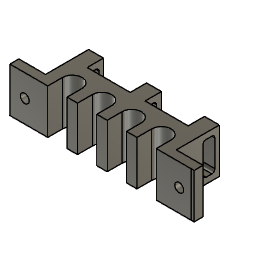
WireClip (Autodesk Fusion 360 design; units mm, degrees)
Autodesk Fusion 360 part; units mm, degrees
sketch "Sketch1" plane through (0, 0, 0) normal (0, 0, 1) x (1, 0, 0)
  line L0 (0, 0) -> (-8, 0)
  line L1 (0, 0) -> (52, 0)
  line L2 (0, 10) -> (44, 10)
  line L3 (44, 10) -> (44, 2)
  line L4 (44, 2) -> (52.000001, 2)
  line L5 (52.000001, 2) -> (52, 0)
  line L6 (-8, 0) -> (-8, 2)
  line L7 (-8, 2) -> (0, 2)
  line L8 (0, 2) -> (0, 10)
  circle A0 centre (7, 5) radius 3.25
  circle A1 centre (17, 5) radius 3.25
  circle A2 centre (37.000001, 5) radius 3.25
  circle A3 centre (27, 5) radius 3.25
  line L9 (7, 5) -> (10.25, 5)
  line L10 (10.25, 5) -> (10.25, -1.628817)
  line L11 (10.25, -1.628817) -> (7, -1.628817)
  line L12 (7, -1.628817) -> (7, 5)
  line L13 (7, 5) -> (3.75, 5)
  line L14 (3.75, 5) -> (3.75, -1.5)
  line L15 (3.75, -1.5) -> (7, -1.5)
  line L16 (7, -1.5) -> (7, 5)
  line L17 (17, 5) -> (20.25, 5)
  line L18 (20.25, 5) -> (20.25, -2)
  line L19 (20.25, -2) -> (17, -2)
  line L20 (17, -2) -> (17, 5)
  line L21 (17, 5) -> (13.75, 5)
  line L22 (13.75, 5) -> (13.75, -3.5)
  line L23 (13.75, -3.5) -> (17, -3.5)
  line L24 (17, -3.5) -> (17, 5)
  line L25 (27, 5) -> (23.75, 5)
  line L26 (23.75, 5) -> (23.75, -2.5)
  line L27 (23.75, -2.5) -> (27, -2.5)
  line L28 (27, -2.5) -> (27, 5)
  line L29 (27, 5) -> (30.25, 5)
  line L30 (30.25, 5) -> (30.25, -3.5)
  line L31 (30.25, -3.5) -> (27, -3.5)
  line L32 (27, -3.5) -> (27, 5)
  line L33 (37.000001, 5) -> (33.750001, 5)
  line L34 (33.750001, 5) -> (33.750001, -1.5)
  line L35 (33.750001, -1.5) -> (37.000001, -1.5)
  line L36 (37.000001, -1.5) -> (37.000001, 5)
  line L37 (37.000001, 5) -> (40.250001, 5)
  line L38 (40.250001, 5) -> (40.250001, -2.5)
  line L39 (40.250001, -2.5) -> (37.000001, -2.5)
  line L40 (37.000001, -2.5) -> (37.000001, 5)
  dimension "d2" = 44
  dimension "d3" = 6.5
  dimension "d4" = 6.5
  dimension "d5" = 6.5
  dimension "d6" = 6.5
  dimension "d9" = 3.25
  dimension "d10" = 3.25
  dimension "d11" = 3.25
  dimension "d12" = 3.25
  constraint coincident L0.start L1.start
  constraint perpendicular L2 L3
  constraint perpendicular L3 L4
  constraint perpendicular L0 L6
  constraint perpendicular L2 L8
  constraint horizontal L9
  constraint vertical L10
  constraint horizontal L11
  constraint vertical L12
  constraint coincident A0.centre L9.start
  constraint horizontal L13
  constraint vertical L14
  constraint horizontal L15
  constraint vertical L16
  constraint horizontal L17
  constraint vertical L18
  constraint horizontal L19
  constraint vertical L20
  constraint coincident A1.centre L17.start
  constraint horizontal L21
  constraint vertical L22
  constraint horizontal L23
  constraint vertical L24
  constraint horizontal L25
  constraint vertical L26
  constraint horizontal L27
  constraint vertical L28
  constraint coincident A3.centre L25.start
  constraint horizontal L29
  constraint vertical L30
  constraint horizontal L31
  constraint vertical L32
  constraint horizontal L33
  constraint vertical L34
  constraint horizontal L35
  constraint vertical L36
  constraint horizontal L37
  constraint vertical L38
  constraint horizontal L39
  constraint vertical L40
  measures "d2" distance of L2.start L2.end
  measures "d3" diameter of A0
  measures "d4" diameter of A1
  measures "d5" diameter of A2
  measures "d6" diameter of A3
  measures "d9" distance of A0.centre L9.end
  measures "d10" distance of A1.centre L17.end
  measures "d11" distance of A3.centre L25.end
sketch "Sketch2" plane through (0, 0, 0) normal (0, 0, 1) x (1, 0, 0)
extrude "Extrude1" add sketch "Sketch1" along normal blind 15 contours L0 L1 L2 L3 L4 L5 L6 L7 L8 A0 A1 A2 A3 L10 L14 L18 L22 L26 L30 L34 L38 picked at (1.2621, 5.828129)
sketch "Sketch3" plane through (0, 2, 0) normal (0, 1, 0) x (-1, 0, 0)
  line L0 (0, 0) -> (8, 0)
  line L1 (8, 0) -> (8, 15)
  line L2 (8, 15) -> (0, 15)
  line L3 (0, 15) -> (0, 0)
  circle A0 centre (4, 7.5) radius 1.5
  circle A1 centre (-48.000001, 7.5) radius 1.5
  dimension "d15" = 3
  dimension "d16" = 3
  measures "d15" diameter of A0
  measures "d16" diameter of A1
extrude "Extrude2" cut sketch "Sketch3" against normal blind 4 contours A0 | A1 picked at (4.091709, 7.857751) picked at (-48.372111, 7.765565)
sketch "Sketch4" plane through (0, 10, 0) normal (0, 1, 0) x (-1, 0, 0)
  line L0 (-44, 0) -> (0, 0)
  line L1 (0, 0) -> (0, 15)
  line L2 (0, 15) -> (-44, 15)
  line L3 (-44, 15) -> (-44, 0)
  line L4 (-5, 0) -> (-5, 15)
  line L5 (-39.000001, 0) -> (-39.000001, 15)
  line L6 (-22, 0) -> (-22, 15)
  line L7 (-22, 12.987575) -> (-19.5, 12.987575)
  line L8 (-19.5, 12.987575) -> (-24.5, 12.987575)
  line L9 (-19.5, 12.987575) -> (-19.5, 15)
  line L10 (-24.5, 12.987575) -> (-24.5, 15)
  line L11 (-19.5, 0) -> (-19.5, 2)
  line L12 (-19.5, 2) -> (-24.5, 2)
  line L13 (-24.5, 2) -> (-24.5, 0)
  line L14 (-5, 12.987575) -> (0, 12.987575)
  line L15 (-5, 2) -> (0, 2)
  line L16 (-39.000001, 13) -> (-44, 13)
  line L17 (-39.000001, 2) -> (-44, 2)
  dimension "d19" = 2.5
  dimension "d20" = 5
  constraint coincident L0 L4.start
  constraint coincident L2 L4.end
  constraint perpendicular L2 L4
  constraint perpendicular L2 L5
  constraint midpoint L0 L6.start
  constraint midpoint L2 L6.end
  constraint perpendicular L6 L7
  constraint perpendicular L6 L8
  constraint coincident L2 L9.end
  constraint perpendicular L2 L9
  constraint coincident L2 L10.end
  constraint perpendicular L2 L10
  constraint coincident L0 L11.start
  constraint perpendicular L0 L11
  constraint perpendicular L6 L12
  constraint coincident L0 L13.end
  constraint perpendicular L12 L13
  constraint perpendicular L1 L14
  constraint coincident L4 L15.start
  constraint coincident L1 L15.end
  constraint perpendicular L1 L15
  constraint coincident L3 L16.end
  constraint perpendicular L3 L16
  constraint coincident L3 L17.end
  constraint perpendicular L3 L17
extrude "Extrude3" add sketch "Sketch4" along normal blind 5 contours L0 L3 L5 L17 | L0 L6 L12 L13 | L2 L3 L5 L16 | L0 L6 L11 L12 | L0 L1 L4 L15 | L2 L6 L8 L10 | L2 L6 L7 L8 L9 | L1 L2 L4 L14 picked at (-42.333334, 1.333333) picked at (-23.666667, 1.333333) picked at (-42.333334, 14.333333) picked at (-21.166667, 1.333333) picked at (-3.333333, 1.333333) picked at (-22.833333, 13.658384) picked at (-21.166667, 14.329192) picked at (-3.333333, 14.329192)
sketch "Sketch5" plane through (0, 0, 12.987575) normal (0, 0, -1) x (1, 0, 0)
  line L0 (24.5, -10) -> (19.5, -10)
  line L1 (19.5, -10) -> (19.5, -15)
  line L2 (19.5, -15) -> (24.5, -15)
  line L3 (24.5, -15) -> (24.5, -10)
  line L4 (24.5, -12.931425) -> (19.5, -12.931425)
  line L5 (5, -10) -> (5, -15)
  line L6 (0, -10) -> (0, -15)
  line L7 (5, -12.931425) -> (0, -12.931425)
  line L8 (39.000001, -12.931425) -> (44.000001, -12.931425)
  constraint perpendicular L1 L4
  constraint perpendicular L1 L7
  constraint perpendicular L6 L8
sketch "Sketch6" plane through (0, 0, 2) normal (0, 0, 1) x (-1, 0, 0)
  line L0 (0, -10) -> (-5, -10)
  line L1 (-5, -10) -> (-5, -15)
  line L2 (-5, -15) -> (0, -15)
  line L3 (0, -15) -> (0, -10)
  line L4 (0, -13) -> (-5, -13)
  line L5 (-19.5, -10) -> (-19.5, -15)
  line L6 (-24.5, -10) -> (-24.5, -15)
  line L7 (-19.5, -13) -> (-24.5, -13)
  line L8 (-39.000001, -10) -> (-39.000001, -15)
  line L9 (-44, -10) -> (-44, -15)
  line L10 (-39.000001, -13) -> (-44.000001, -13)
  constraint coincident L3 L4.start
  constraint coincident L1 L4.end
  constraint perpendicular L1 L4
  constraint coincident L5 L7.start
  constraint coincident L6 L7.end
  constraint perpendicular L1 L7
  constraint perpendicular L6 L10
extrude "Extrude4" add sketch "Sketch5" along normal blind 10.988 contours L1 L2 L3 L4 picked at (21.166667, -13.62095)
sketch "Sketch7" plane through (0, 0, 2) normal (0, 0, 1) x (-1, 0, 0)
  line L0 (-39.000001, -10) -> (-44, -10)
  line L1 (-44, -10) -> (-44, -15)
  line L2 (-44, -15) -> (-39.000001, -15)
  line L3 (-39.000001, -15) -> (-39.000001, -10)
  line L4 (-39.000001, -13) -> (-44.000001, -13)
  point P0 (-39.000001, -13)
  point P1 (-44.000001, -13)
extrude "Extrude5" add sketch "Sketch7" along normal blind 11 contours L1 L2 L3 L4 picked at (-42.333334, -13.666667)
extrude "Extrude6" add sketch "Sketch6" along normal blind 10.988 contours L1 L2 L3 L4 picked at (-3.333333, -13.666667)
extrude "Extrude7" add 1 faces at (52.000001, 1.333333, 5) along direction (1, -0.00000039, 0) blind 1
extrude "Extrude8" add 1 faces at (-8, 0.666667, 5) along direction (-1, 0, 0) blind 1
extrude "Extrude9" add 1 faces at (34.166667, 10, 9.329192) along direction (0, 1, 0) blind 2
extrude "Extrude11" add 3 faces at (3.333333, 15, 5) (21.166667, 15, 10) (42.333334, 15, 5) along direction (0, 1, 0) blind 2.5
extrude "Extrude12" cut 2 faces at (40.666667, 13, 5.666667) (1.666667, 13, 5.662525) along direction (0, 1, 0) blind 3
extrude "Extrude13" cut 1 faces at (22.833333, 12.931425, 9.32505) along direction (0, 1, 0) blind 3
fillet "Fillet3" radius 1 3 edges at (41.500001, 16, 13) (22, 15.931425, 12.987575) (2.5, 16, 12.987575)
fillet "Fillet4" radius 1 3 edges at (2.5, 16, 2) (22, 15.931425, 2) (41.500001, 16, 2)
fillet "Fillet5" radius 1 6 edges at (41.5, 12, 13) (22, 12, 12.987575) (2.5, 12, 12.987575) (2.5, 12, 2) (22, 12, 2) (41.5, 12, 2)
extrude "Extrude14" add 1 faces at (52.333334, 2, 5) along direction (0.00000039, 1, 0) blind 1
extrude "Extrude15" add 1 faces at (47.962635, 2, 2.001398) along direction (0, 1, 0) blind 1
extrude "Extrude16" add 1 faces at (-4.370698, 2, 2.001398) along direction (0, 1, 0) blind 1
equation "d2 = 60 mm - 16 mm"
equation "d9 = ( 6.5 / 2 ) * 1 mm"
equation "d10 = ( 6.5 / 2 ) * 1 mm"
equation "d11 = ( 6.5 / 2 ) * 1 mm"
equation "d12 = ( 6.5 / 2 ) * 1 mm"
